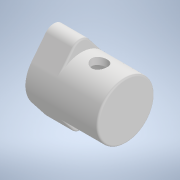
# Autodesk Inventor part: Сборка 13В
Saved by Autodesk Inventor 2021 (Build 250183000, 183)
## iProperties
Created: 2021-03-23
Part Number: Сборка 13В
Material: Типовые
Document SubType Name: Modeling
Designer: khosta
Density: 1 g/cm^3
Appearance: По умолчанию
Author: khosta
Autodesk Inventor part; units mm, degrees
ref_plane "YZ Plane" through (0, 0, 0) normal (1, 0, 0) x (0, 1, 0)
ref_plane "XZ Plane" through (0, 0, 0) normal (0, 1, 0) x (-1, 0, 0)
ref_plane "XY Plane" through (0, 0, 0) normal (0, 0, 1) x (1, 0, 0)
sketch "Эскиз1" plane through (0, 0, 0) normal (1, 0, 0) x (0, 1, 0)
  arc A0 (41.411765, -9.437465) -> (41.411765, 9.437465) centre (34, 0) ccw
  line L0 (20.382353, -25.953029) -> (41.411765, -9.437465)
  line L1 (20.382353, 25.953029) -> (41.411765, 9.437465)
  arc A1 (20.382353, 25.953029) -> (0, 33) centre (0, 0) ccw
  arc A2 (0, -33) -> (20.382353, -25.953029) centre (0, 0) ccw
  arc A3 (-41.411765, 9.437465) -> (-41.411765, -9.437465) centre (-34, 0) ccw
  line L2 (-20.382353, -25.953029) -> (-41.411765, -9.437465)
  line L3 (-20.382353, 25.953029) -> (-41.411765, 9.437465)
  arc A4 (0, 33) -> (-20.382353, 25.953029) centre (0, 0) ccw
  arc A5 (-20.382353, -25.953029) -> (0, -33) centre (0, 0) ccw
  circle A6 centre (0, 0) radius 25
  dimension "d12" = 50
  constraints: 12 point on circle, 8 end point, 7 centre point, 3 tangent, 1 coincident
  measures "d12" diameter of A6
extrude "Выдавливание1" add sketch "Эскиз1" along normal blind 32
sketch "Эскиз2" plane through (32, 0, 0) normal (1, 0, 0) x (0, 0, -1)
  circle A0 centre (0, 0) radius 33
  line L0 (-9.437465, 41.411765) -> (-25.953029, 20.382353)
  circle A1 centre (0, 0) radius 25
  constraints: 2 coincident, 1 centre point, 3 other
extrude "Выдавливание2" add sketch "Эскиз2" along normal blind 45
sketch "Эскиз3" plane through (77, 0, 0) normal (1, 0, 0) x (0, 0, -1)
  circle A0 centre (0, 0) radius 33
  constraints: 1 centre point, 1 coincident
extrude "Выдавливание3" add sketch "Эскиз3" along normal blind 7
sketch "Эскиз4" plane through (0, 0, 0) normal (-1, 0, 0) x (0, 0, 1)
  arc A0 (-9.437465, -41.411765) -> (9.437465, -41.411765) centre (0, -34) ccw
  point P0 (0, 0)
  point P1 (0, 34)
  constraints: 1 coincident
hole "Отверстие1" at (0, -34, 0) at (0, 34, 0) direction (1, 0, 0) diameter 8.917468 depth 23.5 tip angle 120 thread size "M10x1" class "6H" standard "ISO Metric profile"
chamfer "Фаска1" distance 1.6 angle 45 2 edges at (0, 34, -4.4587) (0, -34, -4.4587)
sketch "Эскиз6" plane through (0, 0, 0) normal (0, 1, 0) x (-1, 0, 0)
  line L0 (0, 0) -> (-53, 0)
  circle A0 centre (-53, 0) radius 9
  dimension "d32" = 53
  dimension "d33" = 18
  constraints: 2 end point, 1 centre point, 1 coincident, 1 horizontal
  measures "d32" distance of L0.start L0.end
  measures "d33" diameter of A0
extrude "Выдавливание4" cut sketch "Эскиз6" along normal through all both and the other way through all
fillet "Сопряжение1" radius 2 7 edges at (32, 46, 0) (32, 30.8971, -17.6952) (32, 30.8971, 17.6952) (32, -46, 0) (32, -30.8971, -17.6952) (32, -30.8971, 17.6952) (84, 0, 33)
